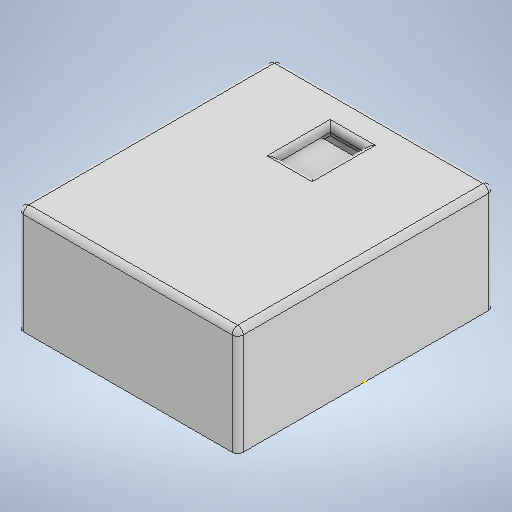
# Autodesk Inventor part: 198MainChassis
Saved by Autodesk Inventor 2025.1 (Build 291241000, 241)
## iProperties
Created: 2024-10-27
Part Number: 198MainChassis
Material: Generic
Document SubType Name: Modeling
Designer: narih
Density: 1 g/cm^3
Appearance: Default
Author: narih
Autodesk Inventor part; units mm, degrees
ref_plane "YZ Plane" through (0, 0, 0) normal (1, 0, 0) x (0, 1, 0)
ref_plane "XZ Plane" through (0, 0, 0) normal (0, 1, 0) x (-1, 0, 0)
ref_plane "XY Plane" through (0, 0, 0) normal (0, 0, 1) x (1, 0, 0)
sketch "Sketch1" plane through (0, 0, 0) normal (0, 1, 0) x (-1, 0, 0)
  line L0 (40.3167, 41.8064) -> (-31.6833, 41.8064)
  line L1 (-31.6833, 41.8064) -> (-31.6833, -43.1936)
  line L2 (-31.6833, -43.1936) -> (40.3167, -43.1936)
  line L3 (40.3167, -43.1936) -> (40.3167, 41.8064)
  line L4 (43.3167, 44.8064) -> (-34.6833, 44.8064)
  line L5 (-34.6833, 44.8064) -> (-34.6833, -46.1936)
  line L6 (-34.6833, -46.1936) -> (43.3167, -46.1936)
  line L7 (43.3167, -46.1936) -> (43.3167, 44.8064)
  point P0 (0, 0)
  dimension "d0" = 85
  dimension "d1" = 72
  dimension "d2" = 3
  dimension "d3" = 3
  dimension "d4" = 3
  dimension "d5" = 3
  constraints: 16 end point, 4 parallel, 2 horizontal, 2 perpendicular
  measures "d0" distance of L2.end L0.start
  measures "d1" distance of L1.end L2.end
  measures "d2" distance between parallel lines of L7 L3
  measures "d3" distance between parallel lines of L6 L2
  measures "d4" distance between parallel lines of L4 L0
  measures "d5" distance between parallel lines of L5 L1
extrude "Extrusion1" add sketch "Sketch1" along normal blind 35
sketch "Sketch2" plane through (0, 35, 0) normal (0, 1, 0) x (1, 0, 0)
  line L0 (34.6833, -44.8064) -> (34.6833, 46.1936) projected
  line L1 (-43.3167, -44.8064) -> (34.6833, -44.8064)
  line L2 (34.6833, -44.8064) -> (34.6833, 46.1936)
  line L3 (34.6833, 46.1936) -> (-43.3167, 46.1936)
  line L4 (-43.3167, 46.1936) -> (-43.3167, -44.8064)
  point P0 (0, 0)
  point P1 (34.6833, -44.8064)
  constraints: 8 end point, 2 parallel, 1 horizontal, 1 perpendicular
extrude "Extrusion2" add sketch "Sketch2" along normal blind 3
sketch "Sketch3" plane through (34.6833, 0, 44.8064) normal (1, 0, 0) x (0, 0, -1)
  point P0 (44.8064, 0)
sketch "Sketch4" plane through (34.6833, 0, -46.1936) normal (0, 0, -1) x (-1, 0, 0)
  circle A0 centre (30.8779, 19.7188) radius 7.0099
  point P0 (34.6833, 0)
  constraints: 1 centre point
extrude "Extrusion3" cut sketch "Sketch4" against normal blind 35
sketch "Sketch5" plane through (0, 38, 0) normal (0, 1, 0) x (1, 0, 0)
  line L0 (-12.108, 16.4323) -> (-0.1673, 16.4323)
  line L1 (-0.1673, 16.4323) -> (-0.1673, 34.8019)
  line L2 (-0.1673, 34.8019) -> (-12.108, 34.8019)
  line L3 (-12.108, 34.8019) -> (-12.108, 16.4323)
  point P0 (0, 0)
  constraints: 8 end point, 2 parallel, 1 horizontal, 1 perpendicular
extrude "Extrusion4" cut sketch "Sketch5" against normal blind 2
sketch "Sketch6" plane through (0, 36, 0) normal (0, 1, 0) x (1, 0, 0)
  point P0 (0, 0)
sketch "Sketch7" plane through (0, 36, 0) normal (0, 1, 0) x (1, 0, 0)
  line L0 (-12.108, 34.8019) -> (-0.1673, 34.8019) projected
  line L1 (-0.1673, 34.8019) -> (-0.1673, 16.4323) projected
  line L2 (-12.108, 34.8019) -> (-0.1673, 34.8019)
  line L3 (-0.1673, 34.8019) -> (-0.1673, 31.7024)
  line L4 (-0.1673, 31.7024) -> (-12.108, 31.7024)
  line L5 (-12.108, 31.7024) -> (-12.108, 34.8019)
  point P0 (0, 0)
  constraints: 8 end point, 2 parallel, 1 horizontal, 1 perpendicular, 1 point on line
extrude "Extrusion5" cut sketch "Sketch7" against normal blind 5
fillet "Fillet1" radius 2 10 edges at (-43.3167, 19, 44.8064) (-43.3167, 19, -46.1936) (-4.3167, 38, -46.1936) (-43.3167, 38, -0.6936) (34.6833, 38, -0.6936) (-6.1377, 38, -16.4323) (-0.1673, 38, -25.6171) (-12.108, 38, -25.6171) (-6.1377, 38, -34.8019) (-4.3167, 38, 44.8064)
fillet "Fillet2" radius 2 4 edges at (34.0975, 37.4142, 44.2206) (34.6833, 18.0001, 44.8064) (34.0975, 37.4142, -45.6079) (34.6833, 18.0001, -46.1936)
fillet "Fillet3" radius 2 1 edges at (10.8153, 19.7188, -46.1936)
body "Solid1"
